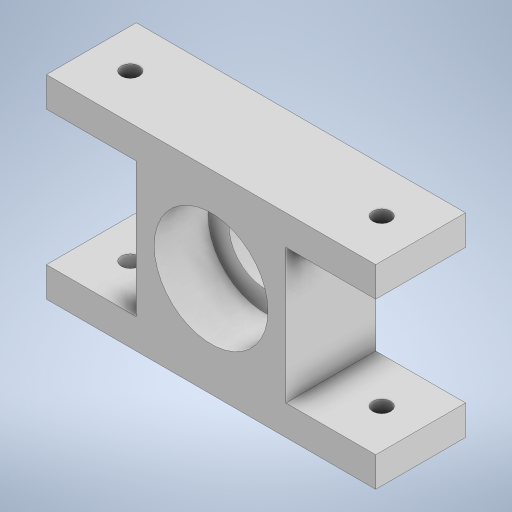
# Autodesk Inventor part: soporte_eje_omni
Saved by Autodesk Inventor 2023.1 (Build 271208000, 208)
## iProperties
Created: 2022-09-07
Part Number: soporte_eje_omni
Material: Genérico
Document SubType Name: Modeling
Designer: Lab. de Manufactura
Density: 1 g/cm^3
Appearance: Valor por defecto
Author: Lab. de Manufactura
## iProperties of the stored document soporte_eje_omni_3DPrint.ipt
Created: 2022-09-08
Part Number: soporte_eje_omni_3DPrint
Material: Genérico
Document SubType Name: Modeling
Designer: Lab. de Manufactura
Density: 1 g/cm^3
Appearance: Valor por defecto
Author: Lab. de Manufactura
Autodesk Inventor part; units mm, degrees
ref_plane "YZ Plane" through (0, 0, 0) normal (1, 0, 0) x (0, 1, 0)
ref_plane "XZ Plane" through (0, 0, 0) normal (0, 1, 0) x (-1, 0, 0)
ref_plane "XY Plane" through (0, 0, 0) normal (0, 0, 1) x (1, 0, 0)
sketch "Boceto1" plane through (0, 0, 0) normal (0, 0, 1) x (1, 0, 0)
  line L0 (-12.5, 16.25) -> (12.5, 16.25)
  line L1 (12.5, 16.25) -> (12.5, -16.25)
  line L2 (12.5, -16.25) -> (-12.5, -16.25)
  line L3 (-12.5, -16.25) -> (-12.5, 16.25)
  line L4 (-12.5, 16.25) -> (12.5, -16.25) construction
  line L5 (12.5, 16.25) -> (-12.5, -16.25) construction
  point P0 (0, 0)
  dimension "d0" = 25
  dimension "d1" = 32.5
  constraints: 12 end point, 2 midpoint, 2 parallel, 1 horizontal, 1 perpendicular
  measures "d0" distance of L0.start L0.end
  measures "d1" distance of L2.end L0.start
extrude "Extrusión1" add sketch "Boceto1" against normal blind 15
sketch "Boceto4" plane through (0, 0, 0) normal (0, 0, 1) x (1, 0, 0)
  circle A0 centre (0, 0.5) radius 9.5
  line L0 (-12.5, -16.25) -> (12.5, -16.25) projected
  line L1 (0, 0) -> (0, 22.8152) construction
  dimension "d20" = 19
  dimension "d21" = 16.75
  constraints: 2 end point, 1 centre point, 1 point on line, 1 vertical
  measures "d20" diameter of A0
  measures "d21" distance from line of L0 A0.centre
extrude "Extrusión4" cut sketch "Boceto4" against normal blind 9
sketch "Boceto5" plane through (0, 0.5, -9) normal (0, 0, 1) x (1, 0, 0)
  circle A0 centre (0, 0) radius 6
  circle A1 centre (0, 0) radius 9.5 projected
  point P0 (0, -0.5)
  point P1 (-7.5, -5.831)
  point P2 (7.5, -5.831)
  dimension "d27" = 12
  constraints: 1 centre point, 1 concentric
  measures "d27" diameter of A0
extrude "Extrusión5" cut sketch "Boceto5" against normal through all contours A0
sketch "Boceto6" plane through (0, 0, -15) normal (0, 0, -1) x (-1, 0, 0)
  line L0 (-12.5, 16.25) -> (-27.5, 16.25)
  line L1 (-27.5, 16.25) -> (-27.5, 11.25)
  line L2 (-27.5, 11.25) -> (-12.5, 11.25)
  line L3 (-12.5, 11.25) -> (-12.5, 16.25)
  line L4 (4.8011, 9.4889) -> (4.8011, -13.0562) construction
  line L5 (0, 15.379) -> (0, -16.25) construction
  line L6 (-12.5, -16.25) -> (12.5, -16.25) projected
  line L7 (12.5, -16.25) -> (12.5, 16.25) construction
  line L8 (12.5, 0) -> (-12.5, 0) construction
  line L9 (-12.5, 16.25) -> (-12.5, -16.25) construction
  line L10 (-12.5, -16.25) -> (-27.5, -16.25)
  line L11 (-27.5, -16.25) -> (-27.5, -11.25)
  line L12 (-27.5, -11.25) -> (-12.5, -11.25)
  line L13 (-12.5, -11.25) -> (-12.5, -16.25)
  line L14 (12.5, 16.25) -> (27.5, 16.25)
  line L15 (27.5, 16.25) -> (27.5, 11.25)
  line L16 (27.5, 11.25) -> (12.5, 11.25)
  line L17 (12.5, 11.25) -> (12.5, 16.25)
  line L18 (12.5, 16.25) -> (12.5, -16.25) construction
  line L19 (12.5, -16.25) -> (27.5, -16.25)
  line L20 (12.5, -11.25) -> (12.5, -16.25)
  line L21 (27.5, -11.25) -> (12.5, -11.25)
  line L22 (27.5, -16.25) -> (27.5, -11.25)
  point P0 (0, 0)
  dimension "d30" = 5
  dimension "d31" = 15
  constraints: 40 end point, 9 symmetric about line, 3 midpoint, 2 parallel, 2 vertical, 1 horizontal, 1 perpendicular
  measures "d30" distance of L0.end L1.end
  measures "d31" distance of L1.end L2.end
extrude "Extrusión6" add sketch "Boceto6" against normal up to surface (15 mm away)
sketch "Boceto8" plane through (-27.5, 16.25, 0) normal (0, 1, 0) x (1, 0, 0)
  line L0 (0, 15) -> (0, 0) construction
  line L1 (0, 7.5) -> (55, 7.5) construction
  line L2 (55, 15) -> (55, 0) construction
  circle A0 centre (6.5, 7.5) radius 1.5
  circle A1 centre (48.5, 7.5) radius 1.5
  line L3 (55, 0) -> (0, 0) projected
  point P0 (27.5, 0)
  point P1 (27.5, 0)
  dimension "d43" = 3
  dimension "d44" = 3
  dimension "d45" = 42
  dimension "d46" = 21
  constraints: 3 midpoint, 2 centre point, 2 end point, 2 point on line
  measures "d43" diameter of A0
  measures "d44" diameter of A1
  measures "d45" distance of A1.centre A0.centre
  measures "d46" horizontal distance of A0.centre point (27.5, 0)
extrude "Extrusión8" cut sketch "Boceto8" against normal through all
